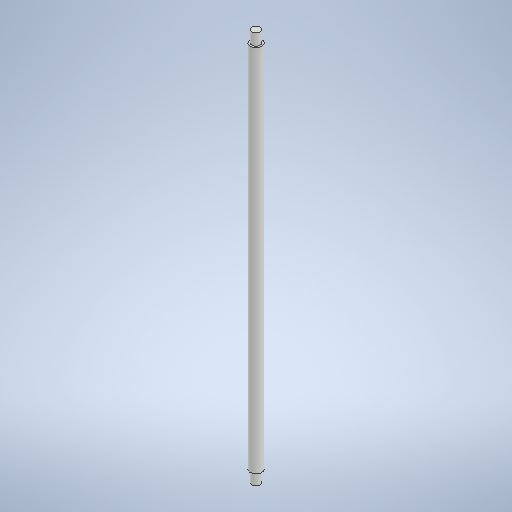
# Autodesk Inventor part: 2071
Saved by Autodesk Inventor 2025.1 (Build 291241000, 241)
## iProperties
Created: 2024-06-10
Part Number: 2071
Material: Generisch
Document SubType Name: Modeling
Designer: ffogue
Density: 1 g/cm^3
Appearance: Vorgabe
Author: ffogue
Autodesk Inventor part; units mm, degrees
ref_plane "YZ Plane" through (0, 0, 0) normal (1, 0, 0) x (0, 1, 0)
ref_plane "XZ Plane" through (0, 0, 0) normal (0, 1, 0) x (-1, 0, 0)
ref_plane "XY Plane" through (0, 0, 0) normal (0, 0, 1) x (1, 0, 0)
sketch "Skizze1" plane through (0, 0, 0) normal (0, 1, 0) x (-1, 0, 0)
  line L0 (0, 0) -> (2.5, 0)
  line L1 (2.5, 0) -> (2.5, -7)
  line L2 (2.5, -7) -> (3.5, -7)
  line L3 (3.5, -7) -> (3.5, -228)
  line L4 (3.5, -228) -> (2.5, -228)
  line L5 (2.5, -228) -> (2.5, -235)
  line L6 (2.5, -235) -> (0, -235)
  line L7 (0, -235) -> (0, 0)
  dimension "d0" = 7
  dimension "d1" = 5
  dimension "d2" = 7
  dimension "d3" = 7
  dimension "d4" = 235
  constraints: 16 end point, 6 perpendicular, 2 point on line, 1 horizontal
  measures "d0" diameter of L3 L7
  measures "d1" diameter of L1 L7
  measures "d2" distance between parallel lines of L6 L4
  measures "d3" distance between parallel lines of L2 L0
  measures "d4" distance between parallel lines of L6 L0
revolve "Umdrehung1" add sketch "Skizze1" angle 360 about axis through (0, 0, -235) along (0, 0, 1)
equation "\"d3\" = d2"
